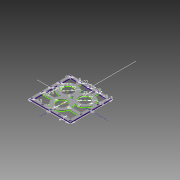
# Autodesk Inventor part: Base
Saved by Autodesk Inventor 2014 SP1 (Build 180222100, 222)
## iProperties
Created: 2015-03-29
Part Number: Base
Material: Generic
Document SubType Name: Modeling
Designer: Erin
Density: 1 g/cm^3
Appearance: Default
Author: Erin
Autodesk Inventor part; units mm, degrees
ref_plane "YZ Plane" through (0, 0, 0) normal (1, 0, 0) x (0, 1, 0)
ref_plane "XZ Plane" through (0, 0, 0) normal (0, 1, 0) x (-1, 0, 0)
ref_plane "XY Plane" through (0, 0, 0) normal (0, 0, 1) x (1, 0, 0)
sketch "Sketch1" plane through (0, 0, 0) normal (0, 0, 1) x (1, 0, 0)
  line L0 (-48, 48) -> (48, 48)
  line L1 (48, 48) -> (48, -48)
  line L2 (48, -48) -> (-48, -48)
  line L3 (-48, -48) -> (-48, 48)
  line L4 (42, 42) -> (-42, 42)
  line L5 (-42, 42) -> (-42, -42)
  line L6 (-42, -42) -> (42, -42)
  line L7 (42, -42) -> (42, 42)
  line L8 (0, 152.7233) -> (0, -72.1628) construction
  line L9 (-77.8847, 0) -> (88.8171, 0) construction
  line L10 (-48, 45) -> (48, 45) construction
  circle A0 centre (0, 45) radius 2.25
  circle A1 centre (-19.75, 45) radius 2.25
  circle A2 centre (19.75, 45) radius 2.25
  line L11 (-45, 48) -> (-45, -48) construction
  circle A3 centre (-45, 45) radius 2.25
  circle A4 centre (-45, 0) radius 2.25
  line L12 (-48, -45) -> (48, -45) construction
  circle A5 centre (-45, -45) radius 2.25
  circle A6 centre (-45, 19.75) radius 2.25
  circle A7 centre (-45, -19.75) radius 2.25
  line L13 (0, -20.208) -> (-19.75, 14) construction
  line L14 (-19.75, 14) -> (19.75, 14) construction
  line L15 (19.75, 14) -> (0, -20.208) construction
  circle A8 centre (19.75, 14) radius 12.5
  circle A9 centre (-19.75, 14) radius 12.5
  circle A10 centre (0, -20.208) radius 12.5
  circle A11 centre (-19.75, 14) radius 20.5
  circle A12 centre (19.75, 14) radius 20.5
  circle A13 centre (0, -20.208) radius 20.5
  line L16 (-23.25, 30.0471) -> (-16.25, 30.0471)
  line L17 (-16.25, 30.0471) -> (-16.25, 42)
  line L18 (-16.25, 42) -> (-23.25, 42)
  line L19 (-23.25, 42) -> (-23.25, 30.0471)
  line L20 (16.25, 30.0471) -> (23.25, 30.0471)
  line L21 (23.25, 30.0471) -> (23.25, 42)
  line L22 (23.25, 42) -> (16.25, 42)
  line L23 (16.25, 42) -> (16.25, 30.0471)
  line L24 (-35.3273, 17.5) -> (-42, 17.5)
  line L25 (-42, 17.5) -> (-42, 10.5)
  line L26 (-42, 10.5) -> (-35.3273, 10.5)
  line L27 (-35.3273, 10.5) -> (-35.3273, 17.5)
  line L28 (34.9738, 17.5) -> (42, 17.5)
  line L29 (42, 17.5) -> (42, 10.5)
  line L30 (42, 10.5) -> (34.9738, 10.5)
  line L31 (34.9738, 10.5) -> (34.9738, 17.5)
  line L32 (-3.5, -36.2367) -> (3.5, -36.2367)
  line L33 (3.5, -36.2367) -> (3.5, -42)
  line L34 (3.5, -42) -> (-3.5, -42)
  line L35 (-3.5, -42) -> (-3.5, -36.2367)
  line L36 (-16.3125, -16.708) -> (-42, -16.708)
  line L37 (-42, -16.708) -> (-42, -23.708)
  line L38 (-42, -23.708) -> (-16.3125, -23.708)
  line L39 (-16.3125, -23.708) -> (-16.3125, -16.708)
  line L40 (16.0929, -16.708) -> (42, -16.708)
  line L41 (42, -16.708) -> (42, -23.708)
  line L42 (42, -23.708) -> (16.0929, -23.708)
  line L43 (16.0929, -23.708) -> (16.0929, -16.708)
  point P0 (0, 0)
  point P1 (0, 48)
  point P2 (48, 0)
  point P3 (0, 2.5973)
  point P4 (-16.3125, -20.208)
  point P5 (16.0929, -20.208)
  point P6 (34.9738, 14)
  point P7 (-35.3273, 14)
  point P8 (-19.75, 30.0471)
  point P9 (19.75, 30.0471)
  point P10 (0, -36.2367)
  dimension "d0" = 96
  dimension "d1" = 96
  dimension "d2" = 6
  dimension "d5" = 3
  dimension "d6" = 4.5
  dimension "d7" = 4.5
  dimension "d8" = 4.5
  dimension "d9" = 22
  dimension "d10" = 22
  dimension "d11" = 3
  dimension "d12" = 4.5
  dimension "d13" = 4.5
  dimension "d14" = 3
  dimension "d15" = 4.5
  dimension "d31" = 4.5
  dimension "d32" = 4.5
  dimension "d33" = 22
  dimension "d34" = 22
  dimension "d53" = 28
  dimension "d54" = 25
  dimension "d55" = 25
  dimension "d56" = 25
  dimension "d65" = 8
  dimension "d66" = 8
  dimension "d67" = 8
  dimension "d68" = 7
  dimension "d69" = 7
  dimension "d70" = 7
  dimension "d71" = 7
  dimension "d72" = 7
  dimension "d73" = 7
  dimension "d74" = 7
  constraints: 88 end point, 23 point on line, 19 parallel, 14 centre point, 13 perpendicular, 11 midpoint, 9 horizontal, 6 coincident, 5 horizontal alignment, 4 vertical alignment, 1 vertical, 10 other
  measures "d0" distance of L1.end L2.end
  measures "d1" distance of L0.end L1.end
  measures "d2" distance between parallel lines of L4 L0
  measures "d5" distance between parallel lines of L10 L0
  measures "d6" diameter of A0
  measures "d7" diameter of A1
  measures "d8" diameter of A2
  measures "d11" distance between parallel lines of L11 L3
  measures "d12" diameter of A3
  measures "d13" diameter of A4
  measures "d14" distance between parallel lines of L12 L2
  measures "d15" diameter of A5
  measures "d31" diameter of A6
  measures "d32" diameter of A7
  measures "d53" distance between parallel lines of L14 L4
  measures "d54" diameter of A8
  measures "d55" diameter of A9
  measures "d56" diameter of A10
  measures "d65" radial gap between concentric circles of A9 A11
  measures "d66" radial gap between concentric circles of A8 A12
  measures "d67" radial gap between concentric circles of A10 A13
  measures "d68" distance of L16.start L16.end
  measures "d69" distance of L20.start L20.end
  measures "d70" distance of L26.end L24.start
  measures "d71" distance of L30.end L28.start
  measures "d72" distance of L38.end L36.start
  measures "d73" distance of L42.end L40.start
  measures "d74" distance of L32.start L32.end
extrude "Extrusion1" add sketch "Sketch1" along normal blind 1.5 contours L0 L1 L2 L3 | L21 A12 L23 L4 | L7 L30 A12 L28 | L21 L20 L23 A12 | A12 L28 L31 L30 A13 A11 L23 L20 L21 | A12 L30 L31 L28 | L17 A11 L19 L4 | L7 L42 A13 L40 | L17 L16 L19 A11 | A11 A12 A13 L26 L27 L24 L19 L16 L17 | A11 A12 | L40 L43 L42 A13 L33 L32 L35 L38 L39 L36 A11 A12 | A13 L42 L43 L40 | A12 A13 | L24 A11 L26 L5 | L24 L27 L26 A11 | A11 A13 | L6 L35 A13 L33 | A13 L35 L32 L33 | L36 A13 L38 L5 | L36 L39 L38 A13 | A0 | A1 | A2 | A3 | A4 | A5 | A6 | A7
extrude "Extrusion2" cut sketch "Sketch1" along normal blind 10 contours A0 | A1 | A2
mirror "Mirror1" about plane through (0, 0, 0) normal (0, 1, 0) of "Extrusion2"
extrude "Extrusion3" cut sketch "Sketch1" along normal blind 10 contours A3 | A4 | A5 | A6 | A7
mirror "Mirror2" about plane through (0, 0, 0) normal (1, 0, 0) of "Extrusion3"
body "Solid1"
